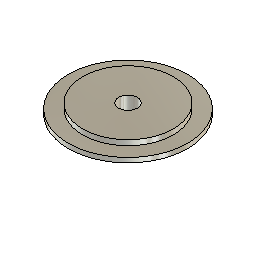
Bottom Rotary Disk v4 (Autodesk Fusion 360 design; units mm, degrees)
Autodesk Fusion 360 part; units mm, degrees
cylinder "CylinderPrimitive1" add diameter 178 height 14.8 placed x (1, 0, 0) y (0, 1, 0) z (0, 0, 1) at (0, 0, 0) makes body 1
sketch "Sketch2" plane through (0, 0, 14.8) normal (0, 0, 1) x (-1, 0, 0)
  circle A0 centre (0, 0) radius 89
  circle A1 centre (0, 0) radius 67.55
  dimension "d3" = 135.1
  constraint concentric A0 A1
  measures "d3" diameter of A1
extrude "Extrude1" cut sketch "Sketch2" against normal blind 7.8 bodies 1
sketch "Sketch3" plane through (0, 0, 14.8) normal (0, 0, 1) x (-1, 0, 0)
  circle A0 centre (0, 0) radius 67.55
  circle A1 centre (0, 0) radius 11.75
  dimension "d6" = 23.5
  constraint coincident A0.centre A1.centre
  measures "d6" diameter of A1
sketch "Sketch4" plane through (0, 0, 0) normal (0, 0, -1) x (1, 0, 0)
  circle A0 centre (0, 0) radius 89
  circle A1 centre (0, 0) radius 24.6
  dimension "d7" = 49.2
  constraint concentric A0 A1
  measures "d7" diameter of A1
extrude "Extrude2" add sketch "Sketch4" along normal blind 11 contours A1 bodies 1
sketch "Sketch5" plane through (0, 0, -11) normal (0, 0, -1) x (1, 0, 0)
  circle A0 centre (0, 0) radius 24.6
  circle A1 centre (0, 0) radius 22.1
  dimension "d10" = 44.2
  constraint coincident A0.centre A1.centre
  measures "d10" diameter of A1
extrude "Extrude3" add sketch "Sketch5" along normal blind 27.5 contours A1 bodies 1
sketch "Sketch6" plane through (0, 0, -38.5) normal (0, 0, -1) x (1, 0, 0)
  circle A0 centre (0, 0) radius 22.1
  circle A1 centre (0, 0) radius 12.65
  dimension "d13" = 25.3
  constraint coincident A0.centre A1.centre
  measures "d13" diameter of A1
extrude "Extrude4" add sketch "Sketch6" along normal blind 12 contours A1 bodies 1
sketch "Sketch9" plane through (0, 0, 0) normal (0, 0, 1) x (1, 0, 0)
  line L0 (100, 160) -> (100, 164.1)
  line L1 (100, 176) -> (100, 171.9)
  line L2 (101.85, 176) -> (100, 176)
  line L3 (101.85, 160) -> (100, 160)
  arc A0 (100, 164.1) -> (100, 171.9) centre (96.8142, 168) ccw
  line L4 (100, 160) -> (105.45, 160)
  line L5 (105.45, 176) -> (101.85, 176)
  line L6 (100, 176) -> (125.6, 176)
  line L7 (125.6, 176) -> (125.6, 160)
  line L8 (125.6, 160) -> (105.45, 160)
  dimension "d16" = 4.1
  dimension "d17" = 16
  dimension "d19" = 4.1
  dimension "d21" = 25.6
  constraint vertical L0
  constraint vertical L1
  constraint horizontal L4
  constraint horizontal L6
  constraint perpendicular L6 L7
  measures "d16" distance of L0.start L0.end
  measures "d17" distance of L0.start L1.start
  measures "d19" distance of L1.start L1.end
  measures "d21" distance of L1.start L6.end
sketch "Sketch10" plane through (0, 176, 0) normal (0, 1, 0) x (-1, 0, 0)
  circle A0 centre (-125.6, 0) radius 25.6
  circle A1 centre (-125.6, 0) radius 22.2
  dimension "d23" = 44.4
  constraint concentric A0 A1
  measures "d23" diameter of A1
copy_body "Body->Comp2" bodies 1 removing the originals makes body 2 in component "plate"
sketch "Sketch11" plane through (0, 0, 14.8) normal (0, 0, 1) x (-1, 0, 0)
  circle A0 centre (0, 0) radius 67.55
  circle A1 centre (0, 0) radius 13.95
  circle A2 centre (0, 0) radius 6
  dimension "d34" = 27.9
  dimension "d35" = 12
  constraint concentric A0 A1
  constraint concentric A1 A2
  measures "d34" diameter of A1
  measures "d35" diameter of A2
extrude "Extrude1'" cut sketch "Sketch11" against normal blind 185 contours A2 bodies 2 in component "plate"
extrude "Extrude2'" cut sketch "Sketch11" against normal blind 25 contours A1 bodies 2 in component "plate"
component "plate" placed x (1, 0, 0) y (0, 1, 0) z (0, 0, 1) at (0, 0, 0)
equation "d21 = ( 51.2 / 2 ) * 1 mm"
